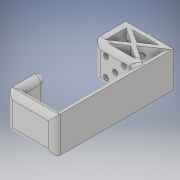
# Autodesk Inventor part: LatexClaw
Saved by Autodesk Inventor 2019 (Build 230136000, 136)
## iProperties
Created: 2018-11-18
Part Number: LatexClaw
Material: Generic
Document SubType Name: Modeling
Designer: mrhftc
Density: 1 g/cm^3
Appearance: Default
Author: mrhftc
Autodesk Inventor part; units mm, degrees
ref_plane "YZ Plane" through (0, 0, 0) normal (1, 0, 0) x (0, 1, 0)
ref_plane "XZ Plane" through (0, 0, 0) normal (0, 1, 0) x (-1, 0, 0)
ref_plane "XY Plane" through (0, 0, 0) normal (0, 0, 1) x (1, 0, 0)
sketch "Sketch1" plane through (0, 0, 0) normal (0, 1, 0) x (-1, 0, 0)
  line L0 (12.7, 63.5) -> (-12.7, 63.5)
  line L1 (-12.7, 63.5) -> (-12.7, 0)
  line L2 (-12.7, 0) -> (12.7, 0)
  line L3 (12.7, 0) -> (12.7, 63.5)
  point P0 (0, 0)
  dimension "d0" = 25.4
  dimension "d1" = 63.5
  constraints: 8 end point, 2 parallel, 1 horizontal, 1 perpendicular
  measures "d0" distance of L1.end L2.end
  measures "d1" distance of L0.end L1.end
extrude "Extrusion1" add sketch "Sketch1" along normal blind 19.05
sketch "Sketch2" plane through (0, 19.05, 0) normal (0, 1, 0) x (1, 0, 0)
  line L0 (-9.5188, -16.8129) -> (9.5312, -16.8129)
  line L1 (9.5312, -16.8129) -> (9.5312, -58.0879)
  line L2 (9.5312, -58.0879) -> (-9.5188, -58.0879)
  line L3 (-9.5188, -58.0879) -> (-9.5188, -16.8129)
  line L4 (12.7, -63.5) -> (12.7, 0) projected
  line L5 (-12.7, 0) -> (-12.7, -63.5) projected
  point P0 (0, 0)
  dimension "d4" = 41.275
  dimension "d5" = 19.05
  dimension "d6" = 3.1688
  dimension "d7" = 3.1812
  constraints: 8 end point, 2 parallel, 1 horizontal, 1 perpendicular
  measures "d4" distance of L2.end L0.start
  measures "d5" distance of L1.end L2.end
  measures "d6" distance between parallel lines of L4 L1
  measures "d7" distance between parallel lines of L5 L3
extrude "Extrusion2" cut sketch "Sketch2" against normal through all
sketch "Sketch3" plane through (0, 19.05, 0) normal (0, 1, 0) x (1, 0, 0)
  point P0 (0, 0)
sketch "Sketch4" plane through (0, 19.05, 0) normal (0, 1, 0) x (1, 0, 0)
  line L0 (-3.7894, -45.3879) -> (-20.6088, -45.3879)
  line L1 (-20.6088, -45.3879) -> (-20.6088, -16.8129)
  line L2 (-20.6088, -16.8129) -> (-3.7894, -16.8129)
  line L3 (-3.7894, -16.8129) -> (-3.7894, -45.3879)
  line L4 (9.5312, -58.0879) -> (-9.5188, -58.0879) projected
  point P0 (0, 0)
  dimension "d10" = 12.7
  dimension "d11" = 28.575
  constraints: 8 end point, 2 parallel, 1 horizontal, 1 perpendicular
  measures "d10" distance between parallel lines of L4 L0
  measures "d11" distance of L0.end L1.end
extrude "Extrusion3" cut sketch "Sketch4" against normal through all
sketch "Sketch5" plane through (-12.7, 0, 0) normal (-1, 0, 0) x (0, 0, 1)
  point P0 (0, 0)
sketch "Sketch6" plane through (0, 19.05, 0) normal (0, 1, 0) x (1, 0, 0)
  line L0 (-12.7, -16.8129) -> (9.5312, -16.8129) projected
  line L1 (-12.7, 0) -> (-12.7, -16.8129) projected
  line L2 (12.7, -63.5) -> (12.7, 0) projected
  line L3 (12.7, 0) -> (-12.7, 0) projected
  line L4 (0.0015, -14.6446) -> (7.0054, -14.6446)
  line L5 (7.0054, -14.6446) -> (0.0015, -9.993)
  line L6 (1.4507, -8.4074) -> (9.5312, -13.878)
  line L7 (9.5312, -13.878) -> (9.5312, -8.4074)
  line L8 (0.0015, -14.6446) -> (-7.0025, -14.6446)
  line L9 (-7.0025, -14.6446) -> (0.0015, -9.993)
  line L10 (-1.4478, -8.4074) -> (-9.5283, -13.878)
  line L11 (-9.5283, -13.878) -> (-9.5283, -8.4074)
  line L12 (0.0015, -2.1702) -> (7.0054, -2.1702)
  line L13 (7.0054, -2.1702) -> (0.0015, -6.8218)
  line L14 (1.4507, -8.4074) -> (9.5312, -2.9368)
  line L15 (9.5312, -2.9368) -> (9.5312, -8.4074)
  line L16 (0.0015, -2.1702) -> (-7.0025, -2.1702)
  line L17 (-7.0025, -2.1702) -> (0.0015, -6.8218)
  line L18 (-1.4478, -8.4074) -> (-9.5283, -2.9368)
  line L19 (-9.5283, -2.9368) -> (-9.5283, -8.4074)
  point P0 (0, 0)
  dimension "d20" = 16.8129
  dimension "d22" = 25.4
  constraints: 32 end point, 1 horizontal
  measures "d20" distance between parallel lines of L3 L0
  measures "d22" distance between parallel lines of L2 L1
extrude "Extrusion5" cut sketch "Sketch6" against normal through all
sketch "Sketch8" plane through (-12.7, 19.05, 16.8129) normal (0, 0, 1) x (1, 0, 0)
  line L0 (22.2312, 0) -> (22.2312, -19.05) projected
  line L1 (22.2312, -9.525) -> (-0.0996, -9.525) construction
  circle A0 centre (11.2604, -9.525) radius 1.3755
  line L2 (11.2604, -9.525) -> (11.5875, -19.05) construction
  line L3 (22.2312, -19.05) -> (0, -19.05) projected
  line L4 (11.2604, -9.525) -> (11.2604, 0) construction
  circle A1 centre (6.3438, -14.4619) radius 1.3755
  circle A2 centre (6.3438, -4.5881) radius 1.3755
  circle A3 centre (16.5041, -14.1131) radius 1.3755
  circle A4 centre (15.8268, -4.2624) radius 1.3755
  point P0 (12.7, -19.05)
  constraints: 6 end point, 5 centre point, 3 symmetric about line, 2 point on line, 1 horizontal, 1 midpoint, 1 vertical, 3 other
extrude "Extrusion6" cut sketch "Sketch8" against normal blind 19.05
fillet "Fillet5" radius 3.175 2 edges at (0.0062, 19.05, 58.0879) (0.0062, 0, 58.0879)
fillet "Fillet8" radius 3.175 1 edges at (-11.1094, 19.05, 45.3879)
fillet "Fillet11" radius 3.175 6 edges at (-11.1094, 0, 45.3879) (-9.5188, 0, 51.7379) (-9.5188, 0, 59.6754) (-1.5844, 0, 16.8129) (-12.7, 9.525, 16.8129) (-1.5844, 19.05, 16.8129)
fillet "Fillet12" radius 3.175 4 edges at (-9.5188, 9.525, 45.3879) (-10.4487, 0.9299, 46.3178) (-9.5188, 19.05, 54.9129) (-9.5188, 18.1201, 46.3178)
fillet "Fillet13" radius 3.175 2 edges at (9.5312, 0, 32.0999) (9.5312, 19.05, 32.0999)
fillet "Fillet14" radius 3.175 3 edges at (10.0039, 1.5082, 16.3402) (10.0039, 17.5418, 16.3402) (9.5312, 9.525, 16.8129)
sketch "Sketch9" plane through (0, 19.05, 0) normal (0, 1, 0) x (1, 0, 0)
  point P0 (0, 0)
fillet "Fillet15" radius 3.175 4 edges at (0, 19.05, 63.5) (-12.7, 9.525, 63.5) (0, 0, 63.5) (12.7, 9.525, 63.5)
body "Solid1"
